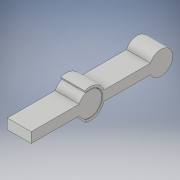
# Autodesk Inventor part: turtlearmJoints
Saved by Autodesk Inventor 2018 (Build 220112000, 112)
## iProperties
Created: 2017-10-25
Part Number: turtlearmJoints
Material: Generic
Document SubType Name: Modeling
Designer: kcmat
Density: 1 g/cm^3
Appearance: Default
Author: kcmat
Autodesk Inventor part; units mm, degrees
ref_plane "YZ Plane" through (0, 0, 0) normal (1, 0, 0) x (0, 1, 0)
ref_plane "XZ Plane" through (0, 0, 0) normal (0, 1, 0) x (-1, 0, 0)
ref_plane "XY Plane" through (0, 0, 0) normal (0, 0, 1) x (1, 0, 0)
sketch "Sketch1" plane through (0, 0, 0) normal (1, 0, 0) x (0, 1, 0)
  circle A0 centre (0, 0) radius 3.175
  line L0 (1.3472, 2.875) -> (1.3472, 15.575)
  line L1 (1.3472, 15.575) -> (-1.3472, 15.575)
  line L2 (-1.3472, 15.575) -> (-1.3472, 2.875)
  arc A1 (1.3472, 2.875) -> (-1.3472, 2.875) centre (0, 0) ccw
  arc A2 (-3.0896, 1.1338) -> (3.0896, 1.1338) centre (0, -0.0687) ccw
  line L3 (-3.0896, 1.1338) -> (-3.3549, 1.1338)
  line L4 (3.0896, 1.1338) -> (3.3102, 1.2365)
  circle A3 centre (-0.026, -18.9035) radius 3.1136
  arc A4 (1.2951, -16.0841) -> (-1.3472, -16.0841) centre (-0.026, -18.9035) ccw
  line L5 (3.0896, 1.1338) -> (3.6653, 1.4017)
  line L6 (-3.0896, 1.1338) -> (-3.7246, 1.1338)
  arc A5 (-3.7246, 1.1338) -> (-1.3472, -3.7376) centre (-0.2877, -0.2047) ccw
  arc A6 (1.2951, -3.7556) -> (3.6653, 1.4017) centre (-0.0687, -0.0056) ccw
  line L7 (1.2951, -3.7556) -> (1.2951, -16.0841)
  line L8 (-1.3472, -16.0841) -> (-1.3472, -3.7376)
  dimension "d0" = 6.35
  dimension "d4" = 12.7
  dimension "d12" = 0.635
  dimension "d13" = 0.635
  constraints: 18 end point, 10 point on circle, 5 centre point, 2 horizontal, 2 parallel, 1 coincident, 8 other
  measures "d4" distance of L0.end L0.start
  measures "d12" distance of L4.start L5.end
  measures "d13" distance of L3.start L6.end
extrude "Extrusion2" add sketch "Sketch1" along normal blind 6.35
body "Solid2"
